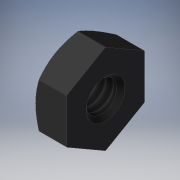
# Autodesk Inventor part: SLBNR2
Saved by Autodesk Inventor 2019 (Build 230136000, 136)
## iProperties
Created: 2024-01-29
Part Number: SLBNR2
Material: Generic
Catalog Web Link: www.cadenas.de
Description: LBNR, LBNL, SLBNR, SLBNL, KNTR, KNTL, SKNTR-Nuts
Vendor: MISUMI
Document SubType Name: Modeling
Designer: psAdmin
Manufacturer: MISUMI
Mass: 0.0187618 g
Surface Area: 0.520817 cm^2
Volume: 0.0187618 cm^3
Density: 1 g/cm^3
Appearance: PSOLRGB-175-175-175
Category: PARTsolutions
Company: MISUMI
Title: SLBNR2
Author: Cadenas PARTsolutions
Comments: Nuts
PSOL_IDENT_0: {$CADENAS_DATA/23d-libs/misumi/metric/27_screws_nuts/slbnl.prj},199 {VTYP=3D},{NB=SLBNR2},{LINA=SLBN
PSOL_IDENT_1: R2},{NN=LBNR, LBNL, SLBNR, SLBNL, KNTR, KNTL, SKNTR},{DATE=03.06.2021 03:35:45},{GEOMDATE=05.11.2010
PSOL_IDENT_2: 00:00:00},{VERSION=},{LINEID=10},{WBVAR=TRS,MAT,CS},{WBNUMERIC=}  {NB=SLBNR2},{LINA=SLBNR2},{KT=DUM
PSOL_IDENT_3: MY},{PN=SLBNR2},{TS=LBN},{TRS=R},{MAT=S},{ST=-},{CS=1},{M1=2},{M=2.0},{P=0.40},{B=4.0},{EE=4.6},{T=1
PSOL_IDENT_4: .6},{T1=0.0},{TFX=1.6},{T1FX=1.2},{CALG='1','JIS Class 1'},{TRSALG= 'R', 'Right-Hand Thread' },{MATA
PSOL_IDENT_5: LG= '', 'SWCH Carbon Steel', 'S', '304 Stainless Steel' }
NB: SLBNR2
NN: LBNR, LBNL, SLBNR, SLBNL, KNTR, KNTL, SKNTR
NT: Nuts
NBSYN: $PN.
LINA: SLBNR2
CATALOG: Misumi
PN: SLBNR2
TRS: Right-Hand Thread
MAT: 304 Stainless Steel Equivalent
ST: -
CS: JIS Class 1
M1: 2
P: 0.4
B: 4
EE: 4.6
T: 1.6
T1: 0
SUPPLIER: MISUMI
ARTICLENO: SLBNR2
BOMINFO: SLBNR2
CREATOR: CADENAS GmbH
Autodesk Inventor part; units mm, degrees
sketch "Sketch_1" plane through (0, 0, 0) normal (0, 0, 1) x (1, 0, 0)
  line L0 (0.8, 0) -> (-0.8, 0)
  line L1 (-0.8, 0) -> (-0.8, 2)
  line L2 (-0.8, 2) -> (-0.6268, 2.3)
  line L3 (-0.6268, 2.3) -> (0.8, 2.3)
  line L4 (0.8, 2.3) -> (0.8, 0)
  line L5 (0.8, 0) -> (-0.8, 0)
  constraints: 12 end point
revolve "Revolution1" add sketch "Sketch_1" angle 360 about axis through (0.8, 0, 0) along (1, 0, 0)
sketch "Sketch_2" plane through (0, 0, 0) normal (0, 0, 1) x (1, 0, 0)
  line L0 (0.8, 0) -> (-0.8, 0)
  line L1 (-0.8, 0) -> (-0.8, 1)
  line L2 (-0.8, 1) -> (-0.5835, 0.7835)
  line L3 (-0.5835, 0.7835) -> (0.5835, 0.7835)
  line L4 (0.5835, 0.7835) -> (0.8, 1)
  line L5 (0.8, 1) -> (0.8, 0)
  line L6 (0.8, 0) -> (-0.8, 0)
  constraints: 14 end point
revolve "Revolution2" cut sketch "Sketch_2" angle 360 about axis through (0.8, 0, 0) along (1, 0, 0)
thread "Thread1" size "M2x0.4" class "6H" standard "ISO Metric profile" full length
sketch "Sketch_3" plane through (0, 0, 0) normal (1, 0, 0) x (0, 1, 0)
  line L0 (-4, 4) -> (-4, -4)
  line L1 (-4, -4) -> (4, -4)
  line L2 (4, -4) -> (4, 4)
  line L3 (4, 4) -> (-4, 4)
  line L4 (-1.1547, 2) -> (-2.3094, 0)
  line L5 (-2.3094, 0) -> (-1.1547, -2)
  line L6 (-1.1547, -2) -> (1.1547, -2)
  line L7 (1.1547, -2) -> (2.3094, 0)
  line L8 (2.3094, 0) -> (1.1547, 2)
  line L9 (1.1547, 2) -> (-1.1547, 2)
  constraints: 20 end point
extrude "Extrusion1" cut sketch "Sketch_3" along normal mid plane 1.6
ref_plane "cp_XY" through (0.8, 0, 0) normal (1, 0, 0) x (0, 0, -1)
ref_plane "cp_YZ" through (0.8, 0, 0) normal (0, 0, -1) x (0, 1, 0)
ref_plane "cp_ZX" through (0.8, 0, 0) normal (0, 1, 0) x (1, 0, 0)
ref_plane "nut_to_screw_XY" through (0, 0, 0) normal (1, 0, 0) x (0, 0, -1)
ref_plane "nut_to_screw_YZ" through (0, 0, 0) normal (0, 0, -1) x (0, 1, 0)
ref_plane "nut_to_screw_ZX" through (0, 0, 0) normal (0, 1, 0) x (1, 0, 0)
body "Solid1"
